Autodesk Fusion 360 part; units mm, degrees
(part 14 of 18)
  spline S14 degree 5 poles (-2.7224, 4.2088) (-2.7224, 4.2088) (-2.7225, 4.209) (-2.7227, 4.2093) (-2.723, 4.2096) (-2.7234, 4.2102) (-2.7238, 4.2109) (-2.7244, 4.2116) (-2.725, 4.2125) (-2.7256, 4.2134) (-2.7263, 4.2144) (-2.7271, 4.2155) (-2.728, 4.2166) (-2.7289, 4.2179) (-2.7299, 4.2192) (-2.7309, 4.2205) (-2.732, 4.222) (-2.7332, 4.2235) (-2.7345, 4.2251) (-2.7358, 4.2267) (-2.7371, 4.2285) (-2.7386, 4.2302) (-2.7401, 4.2321) (-2.7416, 4.234) (-2.7433, 4.236) (-2.7449, 4.238) (-2.7467, 4.2401) (-2.7485, 4.2422) (-2.7504, 4.2444) (-2.7524, 4.2467) (-2.7544, 4.249) (-2.7564, 4.2514) (-2.7586, 4.2538) (-2.7608, 4.2563) (-2.7631, 4.2588) (-2.7654, 4.2613) (-2.7678, 4.264) (-2.7702, 4.2666) (-2.7728, 4.2693) (-2.7754, 4.2721) (-2.778, 4.2749) (-2.7807, 4.2777) (-2.7835, 4.2806) (-2.7863, 4.2835) (-2.7893, 4.2865) (-2.7922, 4.2895) (-2.7953, 4.2925) (-2.7984, 4.2956) (-2.8015, 4.2987) (-2.8047, 4.3019) (-2.808, 4.3051) (-2.8114, 4.3083) (-2.8148, 4.3116) (-2.8182, 4.3149) (-2.8218, 4.3182) (-2.8254, 4.3216) (-2.829, 4.3249) (-2.8328, 4.3284) (-2.8365, 4.3318) (-2.8404, 4.3353) (-2.8443, 4.3388) (-2.8483, 4.3423) (-2.8523, 4.3459) (-2.8564, 4.3495) (-2.8605, 4.3531) (-2.8648, 4.3567) (-2.869, 4.3604) (-2.8734, 4.364) (-2.8778, 4.3678) (-2.8822, 4.3715) (-2.8867, 4.3752) (-2.8913, 4.379) (-2.896, 4.3828) (-2.9007, 4.3866) (-2.9054, 4.3904) (-2.9103, 4.3943) (-2.9152, 4.3981) (-2.9201, 4.402) (-2.9251, 4.4059) (-2.9302, 4.4098) (-2.9353, 4.4138) (-2.9405, 4.4177) (-2.9457, 4.4217) (-2.951, 4.4256) (-2.9564, 4.4296) (-2.9618, 4.4336) (-2.9673, 4.4376) (-2.9728, 4.4416) (-2.9784, 4.4457) (-2.9841, 4.4497) (-2.9898, 4.4538) (-2.9956, 4.4578) (-3.0014, 4.4619) (-3.0073, 4.466) (-3.0133, 4.4701) (-3.0193, 4.4742) (-3.0253, 4.4783) (-3.0314, 4.4824) (-3.0376, 4.4865) (-3.0439, 4.4906) (-3.0502, 4.4948) (-3.0565, 4.4989) (-3.0629, 4.503) (-3.0694, 4.5072) (-3.0759, 4.5113) (-3.0825, 4.5155) (-3.0891, 4.5196) (-3.0958, 4.5238) (-3.1026, 4.5279) (-3.1094, 4.5321) (-3.1162, 4.5362) (-3.1231, 4.5404) (-3.1301, 4.5445) (-3.1371, 4.5487) (-3.1442, 4.5529) (-3.1514, 4.557) (-3.1586, 4.5612) (-3.1658, 4.5653) (-3.1731, 4.5695) (-3.1805, 4.5736) (-3.1879, 4.5777) (-3.1953, 4.5819) (-3.2029, 4.586) (-3.2104, 4.5902) (-3.2181, 4.5943) (-3.2258, 4.5984) (-3.2335, 4.6025) (-3.2413, 4.6066) (-3.2491, 4.6107) (-3.257, 4.6148) (-3.265, 4.6189) (-3.273, 4.623) (-3.281, 4.6271) (-3.2891, 4.6311) (-3.2973, 4.6352) (-3.3055, 4.6392) (-3.3138, 4.6433) (-3.3221, 4.6473) (-3.3304, 4.6513) (-3.3389, 4.6553) (-3.3473, 4.6593) (-3.3559, 4.6633) (-3.3644, 4.6673) (-3.3731, 4.6713) (-3.3817, 4.6752) (-3.3905, 4.6792) (-3.3992, 4.6831) (-3.4081, 4.687) (-3.4169, 4.6909) (-3.4259, 4.6948) (-3.4348, 4.6987) (-3.4439, 4.7026) (-3.4529, 4.7064) (-3.4621, 4.7102) (-3.4712, 4.7141) (-3.4805, 4.7179) (-3.4897, 4.7217) (-3.4991, 4.7254) (-3.5084, 4.7292) (-3.5178, 4.7329) (-3.5273, 4.7367) (-3.5368, 4.7404) (-3.5464, 4.7441) (-3.556, 4.7477) (-3.5657, 4.7514) (-3.5754, 4.755) (-3.5851, 4.7586) (-3.5949, 4.7622) (-3.6048, 4.7658) (-3.6147, 4.7694) (-3.6246, 4.7729) (-3.6346, 4.7765) (-3.6446, 4.78) (-3.6547, 4.7834) (-3.6648, 4.7869) (-3.675, 4.7904) (-3.6852, 4.7938) (-3.6955, 4.7972) (-3.7058, 4.8006) (-3.7161, 4.8039) (-3.7265, 4.8073) (-3.737, 4.8106) (-3.7475, 4.8139) (-3.758, 4.8171) (-3.7686, 4.8204) (-3.7792, 4.8236) (-3.7899, 4.8268) (-3.8006, 4.83) (-3.8113, 4.8331) (-3.8221, 4.8363) (-3.833, 4.8394) (-3.8439, 4.8424) (-3.8548, 4.8455) (-3.8658, 4.8485) (-3.8768, 4.8515) (-3.8878, 4.8545) (-3.8989, 4.8575) (-3.9101, 4.8604) (-3.9212, 4.8633) (-3.9325, 4.8662) (-3.9437, 4.869) (-3.955, 4.8719) (-3.9664, 4.8747) (-3.9778, 4.8774) (-3.9892, 4.8802) (-4.0007, 4.8829) (-4.0122, 4.8856) (-4.0237, 4.8882) (-4.0353, 4.8909) (-4.0469, 4.8935) (-4.0586, 4.896) (-4.0703, 4.8986) (-4.0821, 4.9011) (-4.0939, 4.9036) (-4.1057, 4.906) (-4.1176, 4.9085) (-4.1295, 4.9109) (-4.1414, 4.9132) (-4.1534, 4.9156) (-4.1654, 4.9179) (-4.1775, 4.9201) (-4.1896, 4.9224) (-4.2017, 4.9246) (-4.2139, 4.9268) (-4.2261, 4.9289) (-4.2383, 4.9311) (-4.2506, 4.9332) (-4.2629, 4.9352) (-4.2753, 4.9372) (-4.2877, 4.9392) (-4.3001, 4.9412) (-4.3126, 4.9431) (-4.3251, 4.945) (-4.3377, 4.9469) (-4.3502, 4.9487) (-4.3628, 4.9505) (-4.3755, 4.9523) (-4.3882, 4.954) (-4.4009, 4.9557) (-4.4136, 4.9574) (-4.4264, 4.959) (-4.4367, 4.9603) (-4.4444, 4.9612) (-4.4495, 4.9619) (-4.4521, 4.9622) knots 0 0 0 0 0 0 0.00416667 0.00833333 0.0125 0.01666667 0.02083333 0.025 0.02916667 0.03333333 0.0375 0.04166667 0.04583333 0.05 0.05416667 0.05833333 0.0625 0.06666667 0.07083333 0.075 0.07916667 0.08333333 0.0875 0.09166667 0.09583333 0.1 0.10416667 0.10833333 0.1125 0.11666667 0.12083333 0.125 0.12916667 0.13333333 0.1375 0.14166667 0.14583333 0.15 0.15416667 0.15833333 0.1625 0.16666667 0.17083333 0.175 0.17916667 0.18333333 0.1875 0.19166667 0.19583333 0.2 0.20416667 0.20833333 0.2125 0.21666667 0.22083333 0.225 0.22916667 0.23333333 0.2375 0.24166667 0.24583333 0.25 0.25416667 0.25833333 0.2625 0.26666667 0.27083333 0.275 0.27916667 0.28333333 0.2875 0.29166667 0.29583333 0.3 0.30416667 0.30833333 0.3125 0.31666667 0.32083333 0.325 0.32916667 0.33333333 0.3375 0.34166667 0.34583333 0.35 0.35416667 0.35833333 0.3625 0.36666667 0.37083333 0.375 0.37916667 0.38333333 0.3875 0.39166667 0.39583333 0.4 0.40416667 0.40833333 0.4125 0.41666667 0.42083333 0.425 0.42916667 0.43333333 0.4375 0.44166667 0.44583333 0.45 0.45416667 0.45833333 0.4625 0.46666667 0.47083333 0.475 0.47916667 0.48333333 0.4875 0.49166667 0.49583333 0.5 0.50416667 0.50833333 0.5125 0.51666667 0.52083333 0.525 0.52916667 0.53333333 0.5375 0.54166667 0.54583333 0.55 0.55416667 0.55833333 0.5625 0.56666667 0.57083333 0.575 0.57916667 0.58333333 0.5875 0.59166667 0.59583333 0.6 0.60416667 0.60833333 0.6125 0.61666667 0.62083333 0.625 0.62916667 0.63333333 0.6375 0.64166667 0.64583333 0.65 0.65416667 0.65833333 0.6625 0.66666667 0.67083333 0.675 0.67916667 0.68333333 0.6875 0.69166667 0.69583333 0.7 0.70416667 0.70833333 0.7125 0.71666667 0.72083333 0.725 0.72916667 0.73333333 0.7375 0.74166667 0.74583333 0.75 0.75416667 0.75833333 0.7625 0.76666667 0.77083333 0.775 0.77916667 0.78333333 0.7875 0.79166667 0.79583333 0.8 0.80416667 0.80833333 0.8125 0.81666667 0.82083333 0.825 0.82916667 0.83333333 0.8375 0.84166667 0.84583333 0.85 0.85416667 0.85833333 0.8625 0.86666667 0.87083333 0.875 0.87916667 0.88333333 0.8875 0.89166667 0.89583333 0.9 0.90416667 0.90833333 0.9125 0.91666667 0.92083333 0.925 0.92916667 0.93333333 0.9375 0.94166667 0.94583333 0.95 0.95416667 0.95833333 0.9625 0.96666667 0.97083333 0.975 0.97916667 0.98333333 0.9875 0.99166667 0.99583333 1 1 1 1 1 1
  arc A15 (-4.4521, 4.9622) -> (-4.9622, 4.4521) centre (0, 0) ccw
  spline S15 degree 5 poles (-4.9622, 4.4521) (-4.9619, 4.4495) (-4.9612, 4.4444) (-4.9603, 4.4367) (-4.959, 4.4264) (-4.9574, 4.4136) (-4.9557, 4.4009) (-4.954, 4.3882) (-4.9523, 4.3755) (-4.9505, 4.3628) (-4.9487, 4.3502) (-4.9469, 4.3377) (-4.945, 4.3251) (-4.9431, 4.3126) (-4.9412, 4.3001) (-4.9392, 4.2877) (-4.9372, 4.2753) (-4.9352, 4.2629) (-4.9332, 4.2506) (-4.9311, 4.2383) (-4.9289, 4.2261) (-4.9268, 4.2139) (-4.9246, 4.2017) (-4.9224, 4.1896) (-4.9201, 4.1775) (-4.9179, 4.1654) (-4.9156, 4.1534) (-4.9132, 4.1414) (-4.9109, 4.1295) (-4.9085, 4.1176) (-4.906, 4.1057) (-4.9036, 4.0939) (-4.9011, 4.0821) (-4.8986, 4.0703) (-4.896, 4.0586) (-4.8935, 4.0469) (-4.8909, 4.0353) (-4.8882, 4.0237) (-4.8856, 4.0122) (-4.8829, 4.0007) (-4.8802, 3.9892) (-4.8774, 3.9778) (-4.8747, 3.9664) (-4.8719, 3.955) (-4.869, 3.9437) (-4.8662, 3.9325) (-4.8633, 3.9212) (-4.8604, 3.9101) (-4.8575, 3.8989) (-4.8545, 3.8878) (-4.8515, 3.8768) (-4.8485, 3.8658) (-4.8455, 3.8548) (-4.8424, 3.8439) (-4.8394, 3.833) (-4.8363, 3.8221) (-4.8331, 3.8113) (-4.83, 3.8006) (-4.8268, 3.7899) (-4.8236, 3.7792) (-4.8204, 3.7686) (-4.8171, 3.758) (-4.8139, 3.7475) (-4.8106, 3.737) (-4.8073, 3.7265) (-4.8039, 3.7161) (-4.8006, 3.7058) (-4.7972, 3.6955) (-4.7938, 3.6852) (-4.7904, 3.675) (-4.7869, 3.6648) (-4.7834, 3.6547) (-4.78, 3.6446) (-4.7765, 3.6346) (-4.7729, 3.6246) (-4.7694, 3.6147) (-4.7658, 3.6048) (-4.7622, 3.5949) (-4.7586, 3.5851) (-4.755, 3.5754) (-4.7514, 3.5657) (-4.7477, 3.556) (-4.7441, 3.5464) (-4.7404, 3.5368) (-4.7367, 3.5273) (-4.7329, 3.5178) (-4.7292, 3.5084) (-4.7254, 3.4991) (-4.7217, 3.4897) (-4.7179, 3.4805) (-4.7141, 3.4712) (-4.7102, 3.4621) (-4.7064, 3.4529) (-4.7026, 3.4439) (-4.6987, 3.4348) (-4.6948, 3.4259) (-4.6909, 3.4169) (-4.687, 3.4081) (-4.6831, 3.3992) (-4.6792, 3.3905) (-4.6752, 3.3817) (-4.6713, 3.3731) (-4.6673, 3.3644) (-4.6633, 3.3559) (-4.6593, 3.3473) (-4.6553, 3.3389) (-4.6513, 3.3304) (-4.6473, 3.3221) (-4.6433, 3.3138) (-4.6392, 3.3055) (-4.6352, 3.2973) (-4.6311, 3.2891) (-4.6271, 3.281) (-4.623, 3.273) (-4.6189, 3.265) (-4.6148, 3.257) (-4.6107, 3.2491) (-4.6066, 3.2413) (-4.6025, 3.2335) (-4.5984, 3.2258) (-4.5943, 3.2181) (-4.5902, 3.2104) (-4.586, 3.2029) (-4.5819, 3.1953) (-4.5777, 3.1879) (-4.5736, 3.1805) (-4.5695, 3.1731) (-4.5653, 3.1658) (-4.5612, 3.1586) (-4.557, 3.1514) (-4.5529, 3.1442) (-4.5487, 3.1371) (-4.5445, 3.1301) (-4.5404, 3.1231) (-4.5362, 3.1162) (-4.5321, 3.1094) (-4.5279, 3.1026) (-4.5238, 3.0958) (-4.5196, 3.0891) (-4.5155, 3.0825) (-4.5113, 3.0759) (-4.5072, 3.0694) (-4.503, 3.0629) (-4.4989, 3.0565) (-4.4948, 3.0502) (-4.4906, 3.0439) (-4.4865, 3.0376) (-4.4824, 3.0314) (-4.4783, 3.0253) (-4.4742, 3.0193) (-4.4701, 3.0133) (-4.466, 3.0073) (-4.4619, 3.0014) (-4.4578, 2.9956) (-4.4538, 2.9898) (-4.4497, 2.9841) (-4.4457, 2.9784) (-4.4416, 2.9728) (-4.4376, 2.9673) (-4.4336, 2.9618) (-4.4296, 2.9564) (-4.4256, 2.951) (-4.4217, 2.9457) (-4.4177, 2.9405) (-4.4138, 2.9353) (-4.4098, 2.9302) (-4.4059, 2.9251) (-4.402, 2.9201) (-4.3981, 2.9152) (-4.3943, 2.9103) (-4.3904, 2.9054) (-4.3866, 2.9007) (-4.3828, 2.896) (-4.379, 2.8913) (-4.3752, 2.8867) (-4.3715, 2.8822) (-4.3678, 2.8778) (-4.364, 2.8734) (-4.3604, 2.869) (-4.3567, 2.8648) (-4.3531, 2.8605) (-4.3495, 2.8564) (-4.3459, 2.8523) (-4.3423, 2.8483) (-4.3388, 2.8443) (-4.3353, 2.8404) (-4.3318, 2.8365) (-4.3284, 2.8328) (-4.3249, 2.829) (-4.3216, 2.8254) (-4.3182, 2.8218) (-4.3149, 2.8182) (-4.3116, 2.8148) (-4.3083, 2.8114) (-4.3051, 2.808) (-4.3019, 2.8047) (-4.2987, 2.8015) (-4.2956, 2.7984) (-4.2925, 2.7953) (-4.2895, 2.7922) (-4.2865, 2.7893) (-4.2835, 2.7863) (-4.2806, 2.7835) (-4.2777, 2.7807) (-4.2749, 2.778) (-4.2721, 2.7754) (-4.2693, 2.7728) (-4.2666, 2.7702) (-4.264, 2.7678) (-4.2613, 2.7654) (-4.2588, 2.7631) (-4.2563, 2.7608) (-4.2538, 2.7586) (-4.2514, 2.7564) (-4.249, 2.7544) (-4.2467, 2.7524) (-4.2444, 2.7504) (-4.2422, 2.7485) (-4.2401, 2.7467) (-4.238, 2.7449) (-4.236, 2.7433) (-4.234, 2.7416) (-4.2321, 2.7401) (-4.2302, 2.7386) (-4.2285, 2.7371) (-4.2267, 2.7358) (-4.2251, 2.7345) (-4.2235, 2.7332) (-4.222, 2.732) (-4.2205, 2.7309) (-4.2192, 2.7299) (-4.2179, 2.7289) (-4.2166, 2.728) (-4.2155, 2.7271) (-4.2144, 2.7263) (-4.2134, 2.7256) (-4.2125, 2.725) (-4.2116, 2.7244) (-4.2109, 2.7238) (-4.2102, 2.7234) (-4.2096, 2.723) (-4.2093, 2.7227) (-4.209, 2.7225) (-4.2088, 2.7224) (-4.2088, 2.7224) knots -1 -1 -1 -1 -1 -1 -0.99583333 -0.99166667 -0.9875 -0.98333333 -0.97916667 -0.975 -0.97083333 -0.96666667 -0.9625 -0.95833333 -0.95416667 -0.95 -0.94583333 -0.94166667 -0.9375 -0.93333333 -0.92916667 -0.925 -0.92083333 -0.91666667 -0.9125 -0.90833333 -0.90416667 -0.9 -0.89583333 -0.89166667 -0.8875 -0.88333333 -0.87916667 -0.875 -0.87083333 -0.86666667 -0.8625 -0.85833333 -0.85416667 -0.85 -0.84583333 -0.84166667 -0.8375 -0.83333333 -0.82916667 -0.825 -0.82083333 -0.81666667 -0.8125 -0.80833333 -0.80416667 -0.8 -0.79583333 -0.79166667 -0.7875 -0.78333333 -0.77916667 -0.775 -0.77083333 -0.76666667 -0.7625 -0.75833333 -0.75416667 -0.75 -0.74583333 -0.74166667 -0.7375 -0.73333333 -0.72916667 -0.725 -0.72083333 -0.71666667 -0.7125 -0.70833333 -0.70416667 -0.7 -0.69583333 -0.69166667 -0.6875 -0.68333333 -0.67916667 -0.675 -0.67083333 -0.66666667 -0.6625 -0.65833333 -0.65416667 -0.65 -0.64583333 -0.64166667 -0.6375 -0.63333333 -0.62916667 -0.625 -0.62083333 -0.61666667 -0.6125 -0.60833333 -0.60416667 -0.6 -0.59583333 -0.59166667 -0.5875 -0.58333333 -0.57916667 -0.575 -0.57083333 -0.56666667 -0.5625 -0.55833333 -0.55416667 -0.55 -0.54583333 -0.54166667 -0.5375 -0.53333333 -0.52916667 -0.525 -0.52083333 -0.51666667 -0.5125 -0.50833333 -0.50416667 -0.5 -0.49583333 -0.49166667 -0.4875 -0.48333333 -0.47916667 -0.475 -0.47083333 -0.46666667 -0.4625 -0.45833333 -0.45416667 -0.45 -0.44583333 -0.44166667 -0.4375 -0.43333333 -0.42916667 -0.425 -0.42083333 -0.41666667 -0.4125 -0.40833333 -0.40416667 -0.4 -0.39583333 -0.39166667 -0.3875 -0.38333333 -0.37916667 -0.375 -0.37083333 -0.36666667 -0.3625 -0.35833333 -0.35416667 -0.35 -0.34583333 -0.34166667 -0.3375 -0.33333333 -0.32916667 -0.325 -0.32083333 -0.31666667 -0.3125 -0.30833333 -0.30416667 -0.3 -0.29583333 -0.29166667 -0.2875 -0.28333333 -0.27916667 -0.275 -0.27083333 -0.26666667 -0.2625 -0.25833333 -0.25416667 -0.25 -0.24583333 -0.24166667 -0.2375 -0.23333333 -0.22916667 -0.225 -0.22083333 -0.21666667 -0.2125 -0.20833333 -0.20416667 -0.2 -0.19583333 -0.19166667 -0.1875 -0.18333333 -0.17916667 -0.175 -0.17083333 -0.16666667 -0.1625 -0.15833333 -0.15416667 -0.15 -0.14583333 -0.14166667 -0.1375 -0.13333333 -0.12916667 -0.125 -0.12083333 -0.11666667 -0.1125 -0.10833333 -0.10416667 -0.1 -0.09583333 -0.09166667 -0.0875 -0.08333333 -0.07916667 -0.075 -0.07083333 -0.06666667 -0.0625 -0.05833333 -0.05416667 -0.05 -0.04583333 -0.04166667 -0.0375 -0.03333333 -0.02916667 -0.025 -0.02083333 -0.01666667 -0.0125 -0.00833333 -0.00416667 0 0 0 0 0 0
  line L30 (-4.2088, 2.7224) -> (-4.2081, 2.7219)
  line L31 (-4.2081, 2.7219) -> (-3.0787, 1.9914)
  circle A16 centre (0, 0) radius 2.975
  line L32 (-3, -1) -> (3, -1)
  line L33 (3, -1) -> (3, 1)
  line L34 (3, 1) -> (-3, 1)
  line L35 (-3, 1) -> (-3, -1)
  line L36 (-3, -1) -> (3, 1) construction
  line L37 (3, -1) -> (-3, 1) construction
  line L38 (0.1, -1) -> (0.1, 1)
  line L39 (-2.9, -0.9) -> (2.9, -0.9)
  line L40 (2.9, -0.9) -> (2.9, 0.9)
  line L41 (2.9, 0.9) -> (-2.9, 0.9)
  line L42 (-2.9, 0.9) -> (-2.9, -0.9)
  dimension "d35" = 5.95
  dimension "d38" = -0.1
  constraint coincident A0.centre A1.centre
  constraint horizontal L32
  constraint perpendicular L32 L33
  constraint parallel L32 L34
  constraint parallel L33 L35
  constraint coincident L36 A0.centre
  constraint coincident L37 A0.centre
  constraint coincident L32 L38.start
  constraint coincident L34 L38.end
  constraint perpendicular L34 L38
  measures "d35" diameter of A16
extrude "Extrude3" cut sketch "Sketch4" against normal blind 3 contours A16 L34 L38 L41 | A16 L32 L38 L39 | A16 L34 | A16 L34 L38 L41 | A16 L38 L39 L41 L42 | A16 L32 | A16 L32 L38 L39 | A16 L42 bodies 1 in component "Component"
component "Component" placed x (1, 0, 0) y (0, 1, 0) z (0, 0, 1) at (0, 0, 0)

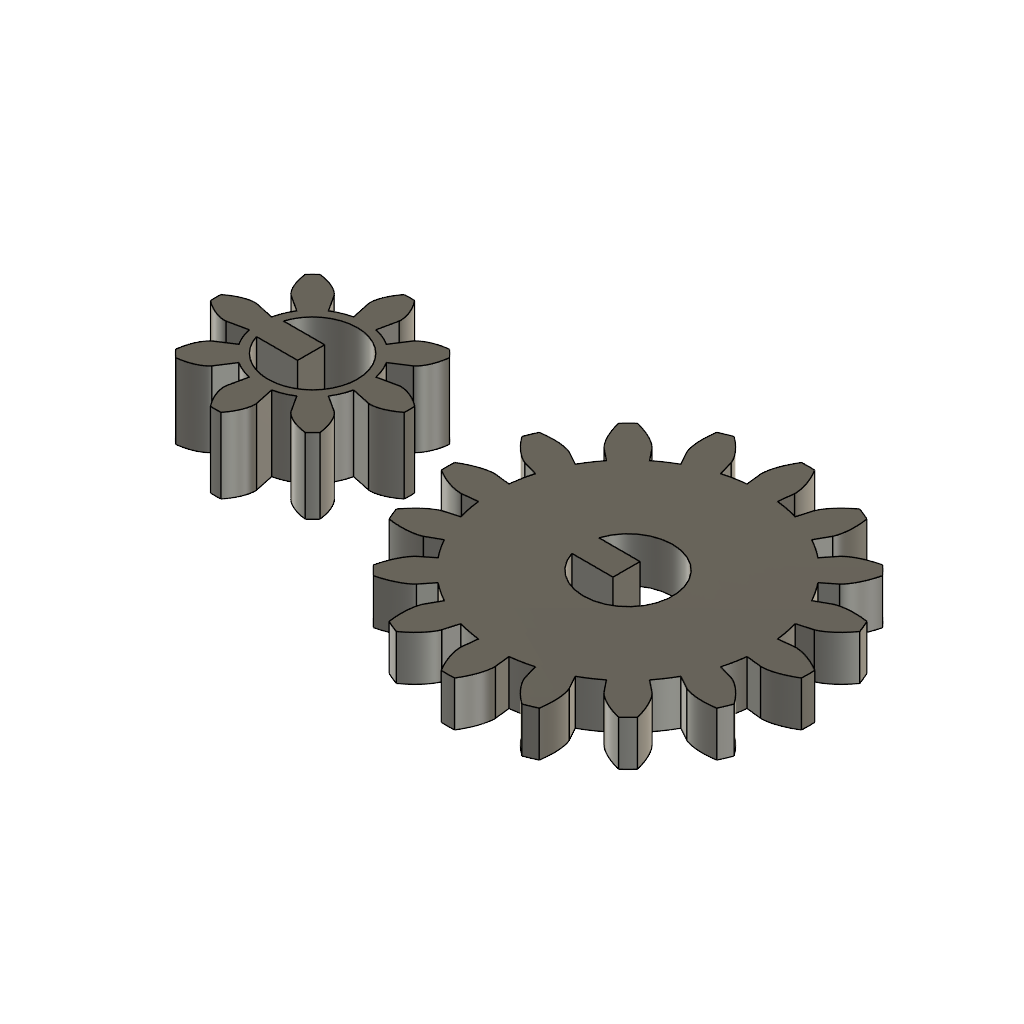
design "card-dispenser-middle-gears"
part number: 2026-09-10-15-09-57-674
part number: 2026-09-10-15-43-32-459
part number: 2026-09-10-16-01-21-363
Autodesk Fusion 360 part; units mm, degrees
sketch "Sketch1" plane through (0, 0, 0) normal (0, 0, 1) x (1, 0, 0) in component "Component"
  spline S0 degree 5 poles (4.747907, -1.018197) (4.747988, -1.018213) (4.748162, -1.018248) (4.748453, -1.018304) (4.748903, -1.018389) (4.749568, -1.01851) (4.750336, -1.018647) (4.751206, -1.018798) (4.752177, -1.018962) (4.753248, -1.019139) (4.754417, -1.019326) (4.755682, -1.019523) (4.757044, -1.019727) (4.758501, -1.019939) (4.760053, -1.020158) (4.761697, -1.020383) (4.763435, -1.020612) (4.765263, -1.020844) (4.767183, -1.02108) (4.769192, -1.021318) (4.771289, -1.021556) (4.773475, -1.021795) (4.775748, -1.022033) (4.778107, -1.02227) (4.780552, -1.022504) (4.783081, -1.022736) (4.785695, -1.022963) (4.788391, -1.023186) (4.79117, -1.023404) (4.79403, -1.023616) (4.796971, -1.023821) (4.799992, -1.024019) (4.803092, -1.024208) (4.806271, -1.024389) (4.809528, -1.024561) (4.812862, -1.024722) (4.816272, -1.024872) (4.819758, -1.025012) (4.82332, -1.025139) (4.826955, -1.025254) (4.830665, -1.025356) (4.834447, -1.025444) (4.838302, -1.025517) (4.842229, -1.025576) (4.846227, -1.02562) (4.850296, -1.025647) (4.854434, -1.025658) (4.858642, -1.025653) (4.862919, -1.025629) (4.867264, -1.025588) (4.871676, -1.025528) (4.876155, -1.025449) (4.8807, -1.025351) (4.885311, -1.025232) (4.889988, -1.025093) (4.894729, -1.024934) (4.899534, -1.024753) (4.904402, -1.02455) (4.909334, -1.024325) (4.914327, -1.024078) (4.919383, -1.023807) (4.9245, -1.023513) (4.929678, -1.023195) (4.934916, -1.022853) (4.940214, -1.022486) (4.945571, -1.022094) (4.950986, -1.021676) (4.95646, -1.021233) (4.961991, -1.020763) (4.96758, -1.020267) (4.973225, -1.019744) (4.978927, -1.019194) (4.984684, -1.018616) (4.990496, -1.01801) (4.996363, -1.017375) (5.002284, -1.016712) (5.008259, -1.01602) (5.014287, -1.015299) (5.020368, -1.014548) (5.026502, -1.013767) (5.032687, -1.012955) (5.038924, -1.012114) (5.045211, -1.011241) (5.051549, -1.010337) (5.057937, -1.009401) (5.064375, -1.008434) (5.070862, -1.007435) (5.077397, -1.006403) (5.083981, -1.005339) (5.090613, -1.004242) (5.097292, -1.003112) (5.104018, -1.001948) (5.110791, -1.000751) (5.117609, -0.99952) (5.124474, -0.998254) (5.131383, -0.996955) (5.138338, -0.99562) (5.145336, -0.994251) (5.152379, -0.992846) (5.159466, -0.991406) (5.166596, -0.98993) (5.173768, -0.988419) (5.180983, -0.986871) (5.18824, -0.985287) (5.195538, -0.983667) (5.202878, -0.98201) (5.210258, -0.980316) (5.217679, -0.978584) (5.22514, -0.976816) (5.23264, -0.97501) (5.24018, -0.973166) (5.247758, -0.971284) (5.255375, -0.969364) (5.263031, -0.967405) (5.270723, -0.965408) (5.278453, -0.963372) (5.28622, -0.961298) (5.294024, -0.959184) (5.301864, -0.957031) (5.30974, -0.954839) (5.317651, -0.952607) (5.325597, -0.950335) (5.333578, -0.948023) (5.341593, -0.945672) (5.349643, -0.943279) (5.357726, -0.940847) (5.365842, -0.938374) (5.373992, -0.93586) (5.382174, -0.933305) (5.390388, -0.930709) (5.398634, -0.928072) (5.406911, -0.925394) (5.41522, -0.922674) (5.42356, -0.919913) (5.43193, -0.917109) (5.44033, -0.914264) (5.448761, -0.911377) (5.45722, -0.908448) (5.465709, -0.905476) (5.474226, -0.902462) (5.482773, -0.899406) (5.491347, -0.896307) (5.499949, -0.893164) (5.508578, -0.88998) (5.517235, -0.886752) (5.525918, -0.88348) (5.534628, -0.880166) (5.543364, -0.876808) (5.552126, -0.873407) (5.560914, -0.869962) (5.569726, -0.866474) (5.578564, -0.862942) (5.587426, -0.859365) (5.596312, -0.855745) (5.605223, -0.852081) (5.614157, -0.848373) (5.623114, -0.84462) (5.632094, -0.840823) (5.641097, -0.836981) (5.650122, -0.833095) (5.659169, -0.829164) (5.668238, -0.825188) (5.677329, -0.821168) (5.686441, -0.817103) (5.695573, -0.812992) (5.704726, -0.808837) (5.713899, -0.804636) (5.723092, -0.800391) (5.732305, -0.7961) (5.741537, -0.791763) (5.750788, -0.787381) (5.760058, -0.782954) (5.769346, -0.778481) (5.778653, -0.773962) (5.787977, -0.769398) (5.797319, -0.764788) (5.806678, -0.760132) (5.816054, -0.75543) (5.825447, -0.750682) (5.834857, -0.745888) (5.844282, -0.741048) (5.853723, -0.736162) (5.86318, -0.73123) (5.872652, -0.726251) (5.882139, -0.721226) (5.891641, -0.716155) (5.901157, -0.711037) (5.910687, -0.705873) (5.920232, -0.700662) (5.929789, -0.695405) (5.93936, -0.690101) (5.948945, -0.684751) (5.958542, -0.679354) (5.968151, -0.67391) (5.977773, -0.66842) (5.987406, -0.662882) (5.997052, -0.657298) (6.006708, -0.651667) (6.016376, -0.645989) (6.026055, -0.640264) (6.035744, -0.634492) (6.045444, -0.628674) (6.055154, -0.622808) (6.064873, -0.616895) (6.074602, -0.610935) (6.084341, -0.604928) (6.094088, -0.598873) (6.103844, -0.592772) (6.113609, -0.586623) (6.123382, -0.580428) (6.133163, -0.574185) (6.142952, -0.567894) (6.152748, -0.561557) (6.162551, -0.555172) (6.172362, -0.54874) (6.182179, -0.54226) (6.192002, -0.535734) (6.201832, -0.52916) (6.211668, -0.522538) (6.221509, -0.515869) (6.231356, -0.509153) (6.241208, -0.50239) (6.251065, -0.495579) (6.260927, -0.48872) (6.270793, -0.481815) (6.280664, -0.474861) (6.290538, -0.467861) (6.300416, -0.460813) (6.310298, -0.453717) (6.320183, -0.446575) (6.330071, -0.439384) (6.339962, -0.432147) (6.349856, -0.424862) (6.359751, -0.417529) (6.369649, -0.410149) (6.379548, -0.402722) (6.389449, -0.395247) (6.399351, -0.387725) (6.409254, -0.380155) (6.419158, -0.372539) (6.429063, -0.364874) (6.436987, -0.358705) (6.442931, -0.354057) (6.446894, -0.350948) (6.448875, -0.349392) knots 0 0 0 0 0 0 0.00416667 0.00833333 0.0125 0.01666667 0.02083333 0.025 0.02916667 0.03333333 0.0375 0.04166667 0.04583333 0.05 0.05416667 0.05833333 0.0625 0.06666667 0.07083333 0.075 0.07916667 0.08333333 0.0875 0.09166667 0.09583333 0.1 0.10416667 0.10833333 0.1125 0.11666667 0.12083333 0.125 0.12916667 0.13333333 0.1375 0.14166667 0.14583333 0.15 0.15416667 0.15833333 0.1625 0.16666667 0.17083333 0.175 0.17916667 0.18333333 0.1875 0.19166667 0.19583333 0.2 0.20416667 0.20833333 0.2125 0.21666667 0.22083333 0.225 0.22916667 0.23333333 0.2375 0.24166667 0.24583333 0.25 0.25416667 0.25833333 0.2625 0.26666667 0.27083333 0.275 0.27916667 0.28333333 0.2875 0.29166667 0.29583333 0.3 0.30416667 0.30833333 0.3125 0.31666667 0.32083333 0.325 0.32916667 0.33333333 0.3375 0.34166667 0.34583333 0.35 0.35416667 0.35833333 0.3625 0.36666667 0.37083333 0.375 0.37916667 0.38333333 0.3875 0.39166667 0.39583333 0.4 0.40416667 0.40833333 0.4125 0.41666667 0.42083333 0.425 0.42916667 0.43333333 0.4375 0.44166667 0.44583333 0.45 0.45416667 0.45833333 0.4625 0.46666667 0.47083333 0.475 0.47916667 0.48333333 0.4875 0.49166667 0.49583333 0.5 0.50416667 0.50833333 0.5125 0.51666667 0.52083333 0.525 0.52916667 0.53333333 0.5375 0.54166667 0.54583333 0.55 0.55416667 0.55833333 0.5625 0.56666667 0.57083333 0.575 0.57916667 0.58333333 0.5875 0.59166667 0.59583333 0.6 0.60416667 0.60833333 0.6125 0.61666667 0.62083333 0.625 0.62916667 0.63333333 0.6375 0.64166667 0.64583333 0.65 0.65416667 0.65833333 0.6625 0.66666667 0.67083333 0.675 0.67916667 0.68333333 0.6875 0.69166667 0.69583333 0.7 0.70416667 0.70833333 0.7125 0.71666667 0.72083333 0.725 0.72916667 0.73333333 0.7375 0.74166667 0.74583333 0.75 0.75416667 0.75833333 0.7625 0.76666667 0.77083333 0.775 0.77916667 0.78333333 0.7875 0.79166667 0.79583333 0.8 0.80416667 0.80833333 0.8125 0.81666667 0.82083333 0.825 0.82916667 0.83333333 0.8375 0.84166667 0.84583333 0.85 0.85416667 0.85833333 0.8625 0.86666667 0.87083333 0.875 0.87916667 0.88333333 0.8875 0.89166667 0.89583333 0.9 0.90416667 0.90833333 0.9125 0.91666667 0.92083333 0.925 0.92916667 0.93333333 0.9375 0.94166667 0.94583333 0.95 0.95416667 0.95833333 0.9625 0.96666667 0.97083333 0.975 0.97916667 0.98333333 0.9875 0.99166667 0.99583333 1 1 1 1 1 1
  spline S1 degree 5 poles (4.747907, 1.018197) (4.747988, 1.018213) (4.748162, 1.018248) (4.748453, 1.018304) (4.748903, 1.018389) (4.749568, 1.01851) (4.750336, 1.018647) (4.751206, 1.018798) (4.752177, 1.018962) (4.753248, 1.019139) (4.754417, 1.019326) (4.755682, 1.019523) (4.757044, 1.019727) (4.758501, 1.019939) (4.760053, 1.020158) (4.761697, 1.020383) (4.763435, 1.020612) (4.765263, 1.020844) (4.767183, 1.02108) (4.769192, 1.021318) (4.771289, 1.021556) (4.773475, 1.021795) (4.775748, 1.022033) (4.778107, 1.02227) (4.780552, 1.022504) (4.783081, 1.022736) (4.785695, 1.022963) (4.788391, 1.023186) (4.79117, 1.023404) (4.79403, 1.023616) (4.796971, 1.023821) (4.799992, 1.024019) (4.803092, 1.024208) (4.806271, 1.024389) (4.809528, 1.024561) (4.812862, 1.024722) (4.816272, 1.024872) (4.819758, 1.025012) (4.82332, 1.025139) (4.826955, 1.025254) (4.830665, 1.025356) (4.834447, 1.025444) (4.838302, 1.025517) (4.842229, 1.025576) (4.846227, 1.02562) (4.850296, 1.025647) (4.854434, 1.025658) (4.858642, 1.025653) (4.862919, 1.025629) (4.867264, 1.025588) (4.871676, 1.025528) (4.876155, 1.025449) (4.8807, 1.025351) (4.885311, 1.025232) (4.889988, 1.025093) (4.894729, 1.024934) (4.899534, 1.024753) (4.904402, 1.02455) (4.909334, 1.024325) (4.914327, 1.024078) (4.919383, 1.023807) (4.9245, 1.023513) (4.929678, 1.023195) (4.934916, 1.022853) (4.940214, 1.022486) (4.945571, 1.022094) (4.950986, 1.021676) (4.95646, 1.021233) (4.961991, 1.020763) (4.96758, 1.020267) (4.973225, 1.019744) (4.978927, 1.019194) (4.984684, 1.018616) (4.990496, 1.01801) (4.996363, 1.017375) (5.002284, 1.016712) (5.008259, 1.01602) (5.014287, 1.015299) (5.020368, 1.014548) (5.026502, 1.013767) (5.032687, 1.012955) (5.038924, 1.012114) (5.045211, 1.011241) (5.051549, 1.010337) (5.057937, 1.009401) (5.064375, 1.008434) (5.070862, 1.007435) (5.077397, 1.006403) (5.083981, 1.005339) (5.090613, 1.004242) (5.097292, 1.003112) (5.104018, 1.001948) (5.110791, 1.000751) (5.117609, 0.99952) (5.124474, 0.998254) (5.131383, 0.996955) (5.138338, 0.99562) (5.145336, 0.994251) (5.152379, 0.992846) (5.159466, 0.991406) (5.166596, 0.98993) (5.173768, 0.988419) (5.180983, 0.986871) (5.18824, 0.985287) (5.195538, 0.983667) (5.202878, 0.98201) (5.210258, 0.980316) (5.217679, 0.978584) (5.22514, 0.976816) (5.23264, 0.97501) (5.24018, 0.973166) (5.247758, 0.971284) (5.255375, 0.969364) (5.263031, 0.967405) (5.270723, 0.965408) (5.278453, 0.963372) (5.28622, 0.961298) (5.294024, 0.959184) (5.301864, 0.957031) (5.30974, 0.954839) (5.317651, 0.952607) (5.325597, 0.950335) (5.333578, 0.948023) (5.341593, 0.945672) (5.349643, 0.943279) (5.357726, 0.940847) (5.365842, 0.938374) (5.373992, 0.93586) (5.382174, 0.933305) (5.390388, 0.930709) (5.398634, 0.928072) (5.406911, 0.925394) (5.41522, 0.922674) (5.42356, 0.919913) (5.43193, 0.917109) (5.44033, 0.914264) (5.448761, 0.911377) (5.45722, 0.908448) (5.465709, 0.905476) (5.474226, 0.902462) (5.482773, 0.899406) (5.491347, 0.896307) (5.499949, 0.893164) (5.508578, 0.88998) (5.517235, 0.886752) (5.525918, 0.88348) (5.534628, 0.880166) (5.543364, 0.876808) (5.552126, 0.873407) (5.560914, 0.869962) (5.569726, 0.866474) (5.578564, 0.862942) (5.587426, 0.859365) (5.596312, 0.855745) (5.605223, 0.852081) (5.614157, 0.848373) (5.623114, 0.84462) (5.632094, 0.840823) (5.641097, 0.836981) (5.650122, 0.833095) (5.659169, 0.829164) (5.668238, 0.825188) (5.677329, 0.821168) (5.686441, 0.817103) (5.695573, 0.812992) (5.704726, 0.808837) (5.713899, 0.804636) (5.723092, 0.800391) (5.732305, 0.7961) (5.741537, 0.791763) (5.750788, 0.787381) (5.760058, 0.782954) (5.769346, 0.778481) (5.778653, 0.773962) (5.787977, 0.769398) (5.797319, 0.764788) (5.806678, 0.760132) (5.816054, 0.75543) (5.825447, 0.750682) (5.834857, 0.745888) (5.844282, 0.741048) (5.853723, 0.736162) (5.86318, 0.73123) (5.872652, 0.726251) (5.882139, 0.721226) (5.891641, 0.716155) (5.901157, 0.711037) (5.910687, 0.705873) (5.920232, 0.700662) (5.929789, 0.695405) (5.93936, 0.690101) (5.948945, 0.684751) (5.958542, 0.679354) (5.968151, 0.67391) (5.977773, 0.66842) (5.987406, 0.662882) (5.997052, 0.657298) (6.006708, 0.651667) (6.016376, 0.645989) (6.026055, 0.640264) (6.035744, 0.634492) (6.045444, 0.628674) (6.055154, 0.622808) (6.064873, 0.616895) (6.074602, 0.610935) (6.084341, 0.604928) (6.094088, 0.598873) (6.103844, 0.592772) (6.113609, 0.586623) (6.123382, 0.580428) (6.133163, 0.574185) (6.142952, 0.567894) (6.152748, 0.561557) (6.162551, 0.555172) (6.172362, 0.54874) (6.182179, 0.54226) (6.192002, 0.535734) (6.201832, 0.52916) (6.211668, 0.522538) (6.221509, 0.515869) (6.231356, 0.509153) (6.241208, 0.50239) (6.251065, 0.495579) (6.260927, 0.48872) (6.270793, 0.481815) (6.280664, 0.474861) (6.290538, 0.467861) (6.300416, 0.460813) (6.310298, 0.453717) (6.320183, 0.446575) (6.330071, 0.439384) (6.339962, 0.432147) (6.349856, 0.424862) (6.359751, 0.417529) (6.369649, 0.410149) (6.379548, 0.402722) (6.389449, 0.395247) (6.399351, 0.387725) (6.409254, 0.380155) (6.419158, 0.372539) (6.429063, 0.364874) (6.436987, 0.358705) (6.442931, 0.354057) (6.446894, 0.350948) (6.448875, 0.349392) knots 0 0 0 0 0 0 0.00416667 0.00833333 0.0125 0.01666667 0.02083333 0.025 0.02916667 0.03333333 0.0375 0.04166667 0.04583333 0.05 0.05416667 0.05833333 0.0625 0.06666667 0.07083333 0.075 0.07916667 0.08333333 0.0875 0.09166667 0.09583333 0.1 0.10416667 0.10833333 0.1125 0.11666667 0.12083333 0.125 0.12916667 0.13333333 0.1375 0.14166667 0.14583333 0.15 0.15416667 0.15833333 0.1625 0.16666667 0.17083333 0.175 0.17916667 0.18333333 0.1875 0.19166667 0.19583333 0.2 0.20416667 0.20833333 0.2125 0.21666667 0.22083333 0.225 0.22916667 0.23333333 0.2375 0.24166667 0.24583333 0.25 0.25416667 0.25833333 0.2625 0.26666667 0.27083333 0.275 0.27916667 0.28333333 0.2875 0.29166667 0.29583333 0.3 0.30416667 0.30833333 0.3125 0.31666667 0.32083333 0.325 0.32916667 0.33333333 0.3375 0.34166667 0.34583333 0.35 0.35416667 0.35833333 0.3625 0.36666667 0.37083333 0.375 0.37916667 0.38333333 0.3875 0.39166667 0.39583333 0.4 0.40416667 0.40833333 0.4125 0.41666667 0.42083333 0.425 0.42916667 0.43333333 0.4375 0.44166667 0.44583333 0.45 0.45416667 0.45833333 0.4625 0.46666667 0.47083333 0.475 0.47916667 0.48333333 0.4875 0.49166667 0.49583333 0.5 0.50416667 0.50833333 0.5125 0.51666667 0.52083333 0.525 0.52916667 0.53333333 0.5375 0.54166667 0.54583333 0.55 0.55416667 0.55833333 0.5625 0.56666667 0.57083333 0.575 0.57916667 0.58333333 0.5875 0.59166667 0.59583333 0.6 0.60416667 0.60833333 0.6125 0.61666667 0.62083333 0.625 0.62916667 0.63333333 0.6375 0.64166667 0.64583333 0.65 0.65416667 0.65833333 0.6625 0.66666667 0.67083333 0.675 0.67916667 0.68333333 0.6875 0.69166667 0.69583333 0.7 0.70416667 0.70833333 0.7125 0.71666667 0.72083333 0.725 0.72916667 0.73333333 0.7375 0.74166667 0.74583333 0.75 0.75416667 0.75833333 0.7625 0.76666667 0.77083333 0.775 0.77916667 0.78333333 0.7875 0.79166667 0.79583333 0.8 0.80416667 0.80833333 0.8125 0.81666667 0.82083333 0.825 0.82916667 0.83333333 0.8375 0.84166667 0.84583333 0.85 0.85416667 0.85833333 0.8625 0.86666667 0.87083333 0.875 0.87916667 0.88333333 0.8875 0.89166667 0.89583333 0.9 0.90416667 0.90833333 0.9125 0.91666667 0.92083333 0.925 0.92916667 0.93333333 0.9375 0.94166667 0.94583333 0.95 0.95416667 0.95833333 0.9625 0.96666667 0.97083333 0.975 0.97916667 0.98333333 0.9875 0.99166667 0.99583333 1 1 1 1 1 1
  spline S2 degree 5 poles (4.747144, -1.018043) (4.747175, -1.018049) (4.747236, -1.018061) (4.747327, -1.01808) (4.747449, -1.018104) (4.747602, -1.018135) (4.747724, -1.01816) (4.747815, -1.018178) (4.747876, -1.01819) (4.747907, -1.018197) knots 0 0 0 0 0 0 0.2 0.4 0.6 0.8 1 1 1 1 1 1
  spline S3 degree 5 poles (4.747144, 1.018043) (4.747175, 1.018049) (4.747236, 1.018061) (4.747327, 1.01808) (4.747449, 1.018104) (4.747602, 1.018135) (4.747724, 1.01816) (4.747815, 1.018178) (4.747876, 1.01819) (4.747907, 1.018197) knots 0 0 0 0 0 0 0.2 0.4 0.6 0.8 1 1 1 1 1 1
  line L0 (0, 0) -> (4.747144, -1.018043)
  line L1 (0, 0) -> (4.747144, 1.018043)
  arc A0 (6.448875, -0.349392) -> (6.448875, 0.349392) centre (0, 0) ccw
  point P0 (4.750201, -1.018622)
  point P1 (4.754038, -1.019265)
  point P2 (4.759424, -1.020069)
  point P3 (4.766367, -1.020979)
  point P4 (4.77487, -1.02194)
  point P5 (4.784939, -1.022896)
  point P6 (4.796574, -1.023791)
  point P7 (4.809777, -1.02457)
  point P8 (4.824547, -1.025176)
  point P9 (4.84088, -1.025554)
  point P10 (4.858773, -1.025648)
  point P11 (4.878221, -1.025402)
  point P12 (4.899217, -1.024761)
  point P13 (4.921752, -1.023668)
  point P14 (4.945817, -1.02207)
  point P15 (4.971399, -1.01991)
  point P16 (4.998487, -1.017134)
  point P17 (5.027066, -1.013688)
  point P18 (5.057119, -1.009517)
  point P19 (5.08863, -1.004567)
  point P20 (5.12158, -0.998785)
  point P21 (5.155949, -0.992117)
  point P22 (5.191714, -0.984512)
  point P23 (5.228854, -0.975918)
  point P24 (5.267344, -0.966282)
  point P25 (5.307157, -0.955554)
  point P26 (5.348266, -0.943683)
  point P27 (5.390644, -0.93062)
  point P28 (5.434259, -0.916316)
  point P29 (5.479081, -0.900722)
  point P30 (5.525077, -0.88379)
  point P31 (5.572213, -0.865475)
  point P32 (5.620453, -0.845729)
  point P33 (5.669762, -0.824508)
  point P34 (5.7201, -0.801767)
  point P35 (5.77143, -0.777463)
  point P36 (5.823711, -0.751553)
  point P37 (5.876901, -0.723996)
  point P38 (5.930958, -0.69475)
  point P39 (5.985838, -0.663777)
  point P40 (6.041495, -0.631037)
  point P41 (6.097885, -0.596494)
  point P42 (6.154959, -0.56011)
  point P43 (6.212669, -0.52185)
  point P44 (6.270967, -0.481681)
  point P45 (6.329802, -0.43957)
  point P46 (6.389122, -0.395483)
  point P47 (4.750201, 1.018622)
  point P48 (4.754038, 1.019265)
  point P49 (4.759424, 1.020069)
  point P50 (4.766367, 1.020979)
  point P51 (4.77487, 1.02194)
  point P52 (4.784939, 1.022896)
  point P53 (4.796574, 1.023791)
  point P54 (4.809777, 1.02457)
  point P55 (4.824547, 1.025176)
  point P56 (4.84088, 1.025554)
  point P57 (4.858773, 1.025648)
  point P58 (4.878221, 1.025402)
  point P59 (4.899217, 1.024761)
  point P60 (4.921752, 1.023668)
  point P61 (4.945817, 1.02207)
  point P62 (4.971399, 1.01991)
  point P63 (4.998487, 1.017134)
  point P64 (5.027066, 1.013688)
  point P65 (5.057119, 1.009517)
  point P66 (5.08863, 1.004567)
  point P67 (5.12158, 0.998785)
  point P68 (5.155949, 0.992117)
  point P69 (5.191714, 0.984512)
  point P70 (5.228854, 0.975918)
  point P71 (5.267344, 0.966282)
  point P72 (5.307157, 0.955554)
  point P73 (5.348266, 0.943683)
  point P74 (5.390644, 0.93062)
  point P75 (5.434259, 0.916316)
  point P76 (5.479081, 0.900722)
  point P77 (5.525077, 0.88379)
  point P78 (5.572213, 0.865475)
  point P79 (5.620453, 0.845729)
  point P80 (5.669762, 0.824508)
  point P81 (5.7201, 0.801767)
  point P82 (5.77143, 0.777463)
  point P83 (5.823711, 0.751553)
  point P84 (5.876901, 0.723996)
  point P85 (5.930958, 0.69475)
  point P86 (5.985838, 0.663777)
  point P87 (6.041495, 0.631037)
  point P88 (6.097885, 0.596494)
  point P89 (6.154959, 0.56011)
  point P90 (6.212669, 0.52185)
  point P91 (6.270967, 0.481681)
  point P92 (6.329802, 0.43957)
  point P93 (6.389122, 0.395483)
sketch "Sketch2" plane through (0, 0, 0) normal (0, 0, 1) x (1, 0, 0) in component "Component"
  circle A0 centre (0, 0) radius 3.552083
extrude "Extrude1" add sketch "Sketch2" along normal blind 3 contours A0 picked at (-0.24006, -0.999023) makes body 1 in component "Component"
extrude "Extrude2" add sketch "Sketch1" along normal blind 3 separate body contours S0 S1 L0 L1 A0 picked at (3.165271, 0) makes body 2 in component "Component"
pattern_circular "C-Pattern1" count 8 over 360 about axis through (0, 0, 1.75) along (0, 0, 1) of "Extrude2" makes body 3 at (1.359084, 0.879101, 1) makes body 4 at (0.339399, 1.582636, 1) makes body 5 at (-0.879101, 1.359084, 1) makes body 6 at (-1.582636, 0.339399, 1) makes body 7 at (-1.359084, -0.879101, 1) makes body 8 at (-0.339399, -1.582636, 1) makes body 9 at (0.879101, -1.359084, 1) in component "Component"
combine "Combine1" operation add target body 1 tool bodies 2 3 4 5 6 7 8 9 in component "Component"
sketch "Sketch3" plane through (0, 0, 0) normal (0, 0, 1) x (1, 0, 0) in component "Component"
  line L0 (0, 0) -> (50.815434, 0) construction
  line L1 (50.815434, 0) -> (50.815434, 3) construction
  line L2 (50.815434, 3) -> (0, 3) construction
  line L3 (0, 3) -> (0, 0) construction
  constraint perpendicular L0 L1
  constraint parallel L0 L2
  constraint parallel L1 L3